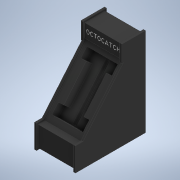
# Autodesk Inventor part: cabinet
Saved by Autodesk Inventor 2020 (Build 240168000, 168)
## iProperties
Created: 2021-03-06
Part Number: cabinet
Material: Generic
Document SubType Name: Modeling
Designer: Harry
Density: 1 g/cm^3
Appearance: Rubber - Black
Author: Harry
Autodesk Inventor part; units mm, degrees
ref_plane "YZ Plane" through (0, 0, 0) normal (1, 0, 0) x (0, 1, 0)
ref_plane "XZ Plane" through (0, 0, 0) normal (0, 1, 0) x (-1, 0, 0)
ref_plane "XY Plane" through (0, 0, 0) normal (0, 0, 1) x (1, 0, 0)
sketch "Sketch1" plane through (0, 0, 0) normal (1, 0, 0) x (0, 1, 0)
  line L0 (0, 0) -> (766.0444, -642.7876)
  line L1 (0, 0) -> (1000, 0) construction
  line L2 (0, 0) -> (0, 100)
  line L3 (0, 100) -> (-300, 100)
  line L4 (-300, 100) -> (-300, -642.7876)
  line L5 (-300, -642.7876) -> (-300, -892.7876)
  line L6 (-300, -892.7876) -> (666.0444, -892.7876)
  line L7 (666.0444, -892.7876) -> (966.0444, -892.7876)
  line L8 (966.0444, -892.7876) -> (966.0444, -592.7876)
  line L9 (966.0444, -592.7876) -> (766.0444, -592.7876)
  line L10 (766.0444, -592.7876) -> (766.0444, -642.7876)
  dimension "d0" = 1000
  dimension "d1" = 40
  dimension "d2" = 100
  dimension "d3" = 300
  dimension "d8" = 250
  dimension "d30" = 200
  dimension "d31" = 300
  constraints: 22 end point, 3 parallel, 2 horizontal, 2 perpendicular, 1 equal length, 1 vertical
  measures "d0" distance of L0.start L0.end
  measures "d1" angle of L0 L1
  measures "d2" distance of L0.start L2.end
  measures "d3" distance of L2.end L3.end
  measures "d8" distance of L4.end L5.end
  measures "d30" distance of L9.end L8.end
  measures "d31" distance of L8.end L7.end
extrude "Extrusion1" add sketch "Sketch1" against normal blind 550
sketch "Sketch3" plane through (-550, 766.0444, -642.7876) normal (0, 0.6427876, 0.7660444) x (1, 0, 0)
  line L0 (0, -1000) -> (0, 0) projected
  line L1 (550, 0) -> (550, -1000) projected
  line L2 (0, 0) -> (550, -1000) construction
  line L3 (550, -1000) -> (0, -1000) projected
  line L4 (0, -1000) -> (550, 0) construction
  line L5 (125, -760) -> (125, -240)
  line L6 (425, -240) -> (425, -760)
  line L7 (425, -760) -> (125, -240) construction
  line L8 (125, -760) -> (425, -240) construction
  line L9 (425, -240) -> (505, -240) construction
  line L10 (45, -240) -> (45, -200)
  line L11 (505, -200) -> (505, -240)
  line L12 (425, -760) -> (505, -760) construction
  line L13 (45, -760) -> (45, -800)
  line L14 (505, -800) -> (505, -760)
  line L15 (505, -760) -> (425, -760)
  line L16 (125, -760) -> (45, -760)
  line L17 (125, -240) -> (132, -240)
  line L18 (418, -240) -> (425, -240)
  line L19 (505, -240) -> (418, -240)
  line L20 (132, -240) -> (45, -240)
  line L21 (505, -800) -> (505, -910)
  line L22 (505, -910) -> (45, -910)
  line L23 (45, -910) -> (45, -800)
  line L24 (505, -200) -> (505, -100)
  line L25 (505, -100) -> (45, -100)
  line L26 (45, -100) -> (45, -200)
  point P0 (275, -500)
  dimension "d9" = 300
  dimension "d10" = 520
  dimension "d11" = 80
  dimension "d12" = 460
  dimension "d13" = 40
  dimension "d14" = 80
  dimension "d15" = 460
  dimension "d16" = 40
  dimension "d21" = 110
  dimension "d22" = 100
  constraints: 48 end point, 6 horizontal, 5 parallel, 4 midpoint, 4 perpendicular, 2 point on line
  measures "d9" distance of L5.end L6.start
  measures "d10" distance of L5.start L5.end
  measures "d11" distance of L6.start L9.end
  measures "d12" distance of L10.end L11.start
  measures "d13" distance of L10.start L10.end
  measures "d14" distance of L6.end L12.end
  measures "d15" distance of L14.start L13.end
  measures "d16" distance of L13.end L13.start
  measures "d21" distance of L21.start L21.end
  measures "d22" distance of L24.end L24.start
extrude "Extrusion3" cut sketch "Sketch3" against normal blind 130
sketch "Sketch4" plane through (-550, 682.4821, -742.3734) normal (0, 0.6427876, 0.7660444) x (1, 0, 0)
  line L0 (125, -760) -> (125, -240) projected
  line L1 (125, -240) -> (425, -760) construction
  line L2 (425, -240) -> (425, -760) projected
  line L3 (125, -760) -> (425, -240) construction
  line L4 (45, -100) -> (505, -100) projected
  line L5 (245, -900) -> (305, -900)
  line L6 (305, -900) -> (305, -100)
  line L7 (305, -100) -> (245, -100)
  line L8 (245, -100) -> (245, -900)
  line L9 (245, -900) -> (305, -100) construction
  line L10 (305, -900) -> (245, -100) construction
  point P0 (550, -1000)
  point P1 (275, -500)
  dimension "d23" = 60
  constraints: 16 end point, 3 midpoint, 2 parallel, 1 horizontal, 1 perpendicular, 1 point on line
  measures "d23" distance of L7.end L6.end
extrude "Extrusion4" cut sketch "Sketch4" against normal blind 60
sketch "Sketch5" plane through (0, 766.0444, -592.7876) normal (0, 0, 1) x (1, 0, 0)
  line L0 (-528.9661, 137.2152) -> (-20.5062, 137.2152) construction
  line L1 (-20.5062, 137.2152) -> (-20.5062, 73.6218) construction
  line L2 (-20.5062, 73.6218) -> (-528.9661, 73.6218) construction
  line L3 (-528.9661, 73.6218) -> (-528.9661, 137.2152) construction
  spline S0 degree 2 poles (-476.9874, 105.246) (-476.9874, 93.0563) (-483.1398, 83.914) knots 0 0 0 1 1 1
  spline S1 degree 2 poles (-483.1398, 83.914) (-489.9246, 73.8518) (-500.5618, 73.8518) knots 0 0 0 1 1 1
  spline S2 degree 2 poles (-500.5618, 73.8518) (-511.1991, 73.8518) (-517.9839, 84.029) knots 0 0 0 1 1 1
  spline S3 degree 2 poles (-517.9839, 84.029) (-524.0787, 93.1713) (-524.0787, 105.246) knots 0 0 0 1 1 1
  spline S4 degree 2 poles (-524.0787, 105.246) (-524.0787, 117.2632) (-518.0414, 126.1755) knots 0 0 0 1 1 1
  spline S5 degree 2 poles (-518.0414, 126.1755) (-510.9691, 136.4677) (-500.5618, 136.4677) knots 0 0 0 1 1 1
  spline S6 degree 2 poles (-500.5618, 136.4677) (-489.4646, 136.4677) (-483.5423, 126.8655) knots 0 0 0 1 1 1
  spline S7 degree 2 poles (-483.5423, 126.8655) (-476.9874, 117.4357) (-476.9874, 105.246) knots 0 0 0 1 1 1
  spline S8 degree 2 poles (-485.7272, 105.246) (-485.7272, 114.2158) (-489.0621, 119.9656) knots 0 0 0 1 1 1
  spline S9 degree 2 poles (-489.0621, 119.9656) (-493.3745, 127.6129) (-500.5618, 127.6129) knots 0 0 0 1 1 1
  spline S10 degree 2 poles (-500.5618, 127.6129) (-507.2892, 127.6129) (-511.5441, 120.4831) knots 0 0 0 1 1 1
  spline S11 degree 2 poles (-511.5441, 120.4831) (-515.339, 114.0433) (-515.339, 105.246) knots 0 0 0 1 1 1
  spline S12 degree 2 poles (-515.339, 105.246) (-515.339, 96.2187) (-513.384, 90.3539) knots 0 0 0 1 1 1
  spline S13 degree 2 poles (-513.384, 90.3539) (-507.5192, 82.7066) (-500.5618, 82.7066) knots 0 0 0 1 1 1
  spline S14 degree 2 poles (-500.5618, 82.7066) (-493.547, 82.7066) (-487.6822, 90.3539) knots 0 0 0 1 1 1
  spline S15 degree 2 poles (-487.6822, 90.3539) (-485.7272, 96.2762) (-485.7272, 105.246) knots 0 0 0 1 1 1
  spline S16 degree 2 poles (-423.3987, 83.914) (-428.3436, 77.9342) (-437.0834, 73.6218) (-443.2358, 73.6218) knots 0 0 0 1 2 2 2
  spline S17 degree 2 poles (-443.2358, 73.6218) (-453.183, 73.6218) (-465.8902, 91.2738) (-465.8902, 105.7635) knots 0 0 0 1 2 2 2
  spline S18 degree 2 poles (-465.8902, 105.7635) (-465.8902, 121.7481) (-458.3004, 130.0279) knots 0 0 0 1 1 1
  spline S19 degree 2 poles (-458.3004, 130.0279) (-452.148, 136.7552) (-443.2358, 136.7552) knots 0 0 0 1 1 1
  spline S20 degree 2 poles (-443.2358, 136.7552) (-436.5659, 136.7552) (-428.1136, 132.0403) (-424.7787, 126.003) knots 0 0 0 1 2 2 2
  spline S21 degree 2 poles (-424.7787, 126.003) (-424.2612, 125.0255) (-424.2612, 123.933) knots 0 0 0 1 1 1
  spline S22 degree 2 poles (-424.2612, 123.933) (-424.2612, 122.1506) (-427.0212, 119.5631) (-428.7461, 119.5631) knots 0 0 0 1 2 2 2
  spline S23 degree 2 poles (-428.7461, 119.5631) (-431.1611, 119.5631) (-432.426, 121.8631) knots 0 0 0 1 1 1
  spline S24 degree 2 poles (-432.426, 121.8631) (-435.8184, 127.9004) (-443.0058, 127.9004) knots 0 0 0 1 1 1
  spline S25 degree 2 poles (-443.0058, 127.9004) (-448.5256, 127.9004) (-452.2055, 123.358) knots 0 0 0 1 1 1
  spline S26 degree 2 poles (-452.2055, 123.358) (-457.0929, 117.2057) (-457.0929, 105.7635) knots 0 0 0 1 1 1
  spline S27 degree 2 poles (-457.0929, 105.7635) (-457.0929, 95.2412) (-448.8706, 82.3616) (-443.0058, 82.3616) knots 0 0 0 1 2 2 2
  spline S28 degree 2 poles (-443.0058, 82.3616) (-435.7034, 82.3616) (-430.8161, 87.5939) knots 0 0 0 1 1 1
  spline S29 degree 2 poles (-430.8161, 87.5939) (-429.2061, 90.9289) (-427.1362, 90.9289) knots 0 0 0 1 1 1
  spline S30 degree 2 poles (-427.1362, 90.9289) (-425.4112, 90.9289) (-422.5363, 88.2264) (-422.5363, 86.3865) knots 0 0 0 1 2 2 2
  spline S31 degree 2 poles (-422.5363, 86.3865) (-422.5363, 84.7765) (-423.3987, 83.914) knots 0 0 0 1 1 1
  line L4 (-370.3276, 127.5554) -> (-385.1622, 127.5554)
  line L5 (-385.1622, 127.5554) -> (-385.1622, 78.2792)
  spline S32 degree 2 poles (-385.1622, 78.2792) (-385.1622, 73.6218) (-389.6471, 73.6218) knots 0 0 0 1 1 1
  spline S33 degree 2 poles (-389.6471, 73.6218) (-394.1895, 73.6218) (-394.1895, 78.2792) knots 0 0 0 1 1 1
  line L6 (-394.1895, 78.2792) -> (-394.1895, 127.5554)
  line L7 (-394.1895, 127.5554) -> (-408.9666, 127.5554)
  spline S34 degree 2 poles (-408.9666, 127.5554) (-413.509, 127.5554) (-413.509, 132.0978) knots 0 0 0 1 1 1
  spline S35 degree 2 poles (-413.509, 132.0978) (-413.509, 136.6402) (-408.9666, 136.6402) knots 0 0 0 1 1 1
  line L8 (-408.9666, 136.6402) -> (-370.3276, 136.6402)
  spline S36 degree 2 poles (-370.3276, 136.6402) (-365.7277, 136.6402) (-365.7277, 132.0978) knots 0 0 0 1 1 1
  spline S37 degree 2 poles (-365.7277, 132.0978) (-365.7277, 127.5554) (-370.3276, 127.5554) knots 0 0 0 1 1 1
  spline S38 degree 2 poles (-310.0691, 105.246) (-310.0691, 93.0563) (-316.2214, 83.914) knots 0 0 0 1 1 1
  spline S39 degree 2 poles (-316.2214, 83.914) (-323.0062, 73.8518) (-333.6435, 73.8518) knots 0 0 0 1 1 1
  spline S40 degree 2 poles (-333.6435, 73.8518) (-344.2807, 73.8518) (-351.0655, 84.029) knots 0 0 0 1 1 1
  spline S41 degree 2 poles (-351.0655, 84.029) (-357.1604, 93.1713) (-357.1604, 105.246) knots 0 0 0 1 1 1
  spline S42 degree 2 poles (-357.1604, 105.246) (-357.1604, 117.2632) (-351.123, 126.1755) knots 0 0 0 1 1 1
  spline S43 degree 2 poles (-351.123, 126.1755) (-344.0507, 136.4677) (-333.6435, 136.4677) knots 0 0 0 1 1 1
  spline S44 degree 2 poles (-333.6435, 136.4677) (-322.5463, 136.4677) (-316.6239, 126.8655) knots 0 0 0 1 1 1
  spline S45 degree 2 poles (-316.6239, 126.8655) (-310.0691, 117.4357) (-310.0691, 105.246) knots 0 0 0 1 1 1
  spline S46 degree 2 poles (-318.8088, 105.246) (-318.8088, 114.2158) (-322.1438, 119.9656) knots 0 0 0 1 1 1
  spline S47 degree 2 poles (-322.1438, 119.9656) (-326.4562, 127.6129) (-333.6435, 127.6129) knots 0 0 0 1 1 1
  spline S48 degree 2 poles (-333.6435, 127.6129) (-340.3708, 127.6129) (-344.6257, 120.4831) knots 0 0 0 1 1 1
  spline S49 degree 2 poles (-344.6257, 120.4831) (-348.4206, 114.0433) (-348.4206, 105.246) knots 0 0 0 1 1 1
  spline S50 degree 2 poles (-348.4206, 105.246) (-348.4206, 96.2187) (-346.4657, 90.3539) knots 0 0 0 1 1 1
  spline S51 degree 2 poles (-346.4657, 90.3539) (-340.6008, 82.7066) (-333.6435, 82.7066) knots 0 0 0 1 1 1
  spline S52 degree 2 poles (-333.6435, 82.7066) (-326.6287, 82.7066) (-320.7638, 90.3539) knots 0 0 0 1 1 1
  spline S53 degree 2 poles (-320.7638, 90.3539) (-318.8088, 96.2762) (-318.8088, 105.246) knots 0 0 0 1 1 1
  spline S54 degree 2 poles (-256.4804, 83.914) (-261.4253, 77.9342) (-270.1651, 73.6218) (-276.3174, 73.6218) knots 0 0 0 1 2 2 2
  spline S55 degree 2 poles (-276.3174, 73.6218) (-286.2647, 73.6218) (-298.9718, 91.2738) (-298.9718, 105.7635) knots 0 0 0 1 2 2 2
  spline S56 degree 2 poles (-298.9718, 105.7635) (-298.9718, 121.7481) (-291.382, 130.0279) knots 0 0 0 1 1 1
  spline S57 degree 2 poles (-291.382, 130.0279) (-285.2297, 136.7552) (-276.3174, 136.7552) knots 0 0 0 1 1 1
  spline S58 degree 2 poles (-276.3174, 136.7552) (-269.6476, 136.7552) (-261.1953, 132.0403) (-257.8604, 126.003) knots 0 0 0 1 2 2 2
  spline S59 degree 2 poles (-257.8604, 126.003) (-257.3429, 125.0255) (-257.3429, 123.933) knots 0 0 0 1 1 1
  spline S60 degree 2 poles (-257.3429, 123.933) (-257.3429, 122.1506) (-260.1028, 119.5631) (-261.8278, 119.5631) knots 0 0 0 1 2 2 2
  spline S61 degree 2 poles (-261.8278, 119.5631) (-264.2427, 119.5631) (-265.5077, 121.8631) knots 0 0 0 1 1 1
  spline S62 degree 2 poles (-265.5077, 121.8631) (-268.9001, 127.9004) (-276.0874, 127.9004) knots 0 0 0 1 1 1
  spline S63 degree 2 poles (-276.0874, 127.9004) (-281.6073, 127.9004) (-285.2872, 123.358) knots 0 0 0 1 1 1
  spline S64 degree 2 poles (-285.2872, 123.358) (-290.1746, 117.2057) (-290.1746, 105.7635) knots 0 0 0 1 1 1
  spline S65 degree 2 poles (-290.1746, 105.7635) (-290.1746, 95.2412) (-281.9523, 82.3616) (-276.0874, 82.3616) knots 0 0 0 1 2 2 2
  spline S66 degree 2 poles (-276.0874, 82.3616) (-268.7851, 82.3616) (-263.8977, 87.5939) knots 0 0 0 1 1 1
  spline S67 degree 2 poles (-263.8977, 87.5939) (-262.2877, 90.9289) (-260.2178, 90.9289) knots 0 0 0 1 1 1
  spline S68 degree 2 poles (-260.2178, 90.9289) (-258.4928, 90.9289) (-255.6179, 88.2264) (-255.6179, 86.3865) knots 0 0 0 1 2 2 2
  spline S69 degree 2 poles (-255.6179, 86.3865) (-255.6179, 84.7765) (-256.4804, 83.914) knots 0 0 0 1 1 1
  spline S70 degree 2 poles (-193.8644, 79.8316) (-193.577, 78.9692) (-193.577, 78.1642) knots 0 0 0 1 1 1
  spline S71 degree 2 poles (-193.577, 78.1642) (-193.577, 76.2667) (-196.4519, 73.8518) (-198.1768, 73.8518) knots 0 0 0 1 2 2 2
  spline S72 degree 2 poles (-198.1768, 73.8518) (-201.1093, 73.8518) (-202.0867, 76.6117) knots 0 0 0 1 1 1
  line L9 (-202.0867, 76.6117) -> (-205.6517, 85.294)
  line L10 (-205.6517, 85.294) -> (-233.711, 85.294)
  line L11 (-233.711, 85.294) -> (-236.9884, 76.6692)
  spline S73 degree 2 poles (-236.9884, 76.6692) (-238.1958, 73.8518) (-241.1283, 73.8518) knots 0 0 0 1 1 1
  spline S74 degree 2 poles (-241.1283, 73.8518) (-245.5557, 73.8518) (-245.5557, 78.1067) knots 0 0 0 1 1 1
  spline S75 degree 2 poles (-245.5557, 78.1067) (-245.5557, 78.9117) (-245.3257, 79.6016) knots 0 0 0 1 1 1
  line L12 (-245.3257, 79.6016) -> (-224.5112, 134.5128)
  spline S76 degree 2 poles (-224.5112, 134.5128) (-222.7287, 137.2152) (-220.0838, 137.2152) knots 0 0 0 1 1 1
  spline S77 degree 2 poles (-220.0838, 137.2152) (-217.4389, 137.2152) (-215.5989, 134.5703) knots 0 0 0 1 1 1
  line L13 (-215.5989, 134.5703) -> (-193.8644, 79.8316)
  line L14 (-208.5841, 94.0338) -> (-219.9688, 123.9905)
  line L15 (-219.9688, 123.9905) -> (-231.0085, 94.0338)
  line L16 (-231.0085, 94.0338) -> (-208.5841, 94.0338)
  line L17 (-139.8733, 127.5554) -> (-154.7079, 127.5554)
  line L18 (-154.7079, 127.5554) -> (-154.7079, 78.2792)
  spline S78 degree 2 poles (-154.7079, 78.2792) (-154.7079, 73.6218) (-159.1928, 73.6218) knots 0 0 0 1 1 1
  spline S79 degree 2 poles (-159.1928, 73.6218) (-163.7352, 73.6218) (-163.7352, 78.2792) knots 0 0 0 1 1 1
  line L19 (-163.7352, 78.2792) -> (-163.7352, 127.5554)
  line L20 (-163.7352, 127.5554) -> (-178.5123, 127.5554)
  spline S80 degree 2 poles (-178.5123, 127.5554) (-183.0547, 127.5554) (-183.0547, 132.0978) knots 0 0 0 1 1 1
  spline S81 degree 2 poles (-183.0547, 132.0978) (-183.0547, 136.6402) (-178.5123, 136.6402) knots 0 0 0 1 1 1
  line L21 (-178.5123, 136.6402) -> (-139.8733, 136.6402)
  spline S82 degree 2 poles (-139.8733, 136.6402) (-135.2734, 136.6402) (-135.2734, 132.0978) knots 0 0 0 1 1 1
  spline S83 degree 2 poles (-135.2734, 132.0978) (-135.2734, 127.5554) (-139.8733, 127.5554) knots 0 0 0 1 1 1
  spline S84 degree 2 poles (-82.3172, 83.914) (-87.2621, 77.9342) (-96.0019, 73.6218) (-102.1542, 73.6218) knots 0 0 0 1 2 2 2
  spline S85 degree 2 poles (-102.1542, 73.6218) (-112.1015, 73.6218) (-124.8087, 91.2738) (-124.8087, 105.7635) knots 0 0 0 1 2 2 2
  spline S86 degree 2 poles (-124.8087, 105.7635) (-124.8087, 121.7481) (-117.2189, 130.0279) knots 0 0 0 1 1 1
  spline S87 degree 2 poles (-117.2189, 130.0279) (-111.0665, 136.7552) (-102.1542, 136.7552) knots 0 0 0 1 1 1
  spline S88 degree 2 poles (-102.1542, 136.7552) (-95.4844, 136.7552) (-87.0321, 132.0403) (-83.6972, 126.003) knots 0 0 0 1 2 2 2
  spline S89 degree 2 poles (-83.6972, 126.003) (-83.1797, 125.0255) (-83.1797, 123.933) knots 0 0 0 1 1 1
  spline S90 degree 2 poles (-83.1797, 123.933) (-83.1797, 122.1506) (-85.9396, 119.5631) (-87.6646, 119.5631) knots 0 0 0 1 2 2 2
  spline S91 degree 2 poles (-87.6646, 119.5631) (-90.0795, 119.5631) (-91.3445, 121.8631) knots 0 0 0 1 1 1
  spline S92 degree 2 poles (-91.3445, 121.8631) (-94.7369, 127.9004) (-101.9242, 127.9004) knots 0 0 0 1 1 1
  spline S93 degree 2 poles (-101.9242, 127.9004) (-107.4441, 127.9004) (-111.124, 123.358) knots 0 0 0 1 1 1
  spline S94 degree 2 poles (-111.124, 123.358) (-116.0114, 117.2057) (-116.0114, 105.7635) knots 0 0 0 1 1 1
  spline S95 degree 2 poles (-116.0114, 105.7635) (-116.0114, 95.2412) (-107.7891, 82.3616) (-101.9242, 82.3616) knots 0 0 0 1 2 2 2
  spline S96 degree 2 poles (-101.9242, 82.3616) (-94.6219, 82.3616) (-89.7345, 87.5939) knots 0 0 0 1 1 1
  spline S97 degree 2 poles (-89.7345, 87.5939) (-88.1246, 90.9289) (-86.0546, 90.9289) knots 0 0 0 1 1 1
  spline S98 degree 2 poles (-86.0546, 90.9289) (-84.3297, 90.9289) (-81.4547, 88.2264) (-81.4547, 86.3865) knots 0 0 0 1 2 2 2
  spline S99 degree 2 poles (-81.4547, 86.3865) (-81.4547, 84.7765) (-82.3172, 83.914) knots 0 0 0 1 1 1
  spline S100 degree 2 poles (-26.6586, 78.3942) (-26.6586, 73.8518) (-31.0285, 73.8518) knots 0 0 0 1 1 1
  spline S101 degree 2 poles (-31.0285, 73.8518) (-35.4559, 73.8518) (-35.4559, 78.3942) knots 0 0 0 1 1 1
  line L22 (-35.4559, 78.3942) -> (-35.4559, 102.7736)
  line L23 (-35.4559, 102.7736) -> (-61.3877, 102.7736)
  line L24 (-61.3877, 102.7736) -> (-61.3877, 78.3942)
  spline S102 degree 2 poles (-61.3877, 78.3942) (-61.3877, 73.8518) (-65.8726, 73.8518) knots 0 0 0 1 1 1
  spline S103 degree 2 poles (-65.8726, 73.8518) (-70.3, 73.8518) (-70.3, 78.3942) knots 0 0 0 1 1 1
  line L25 (-70.3, 78.3942) -> (-70.3, 132.2128)
  spline S104 degree 2 poles (-70.3, 132.2128) (-70.3, 136.7552) (-65.8726, 136.7552) knots 0 0 0 1 1 1
  spline S105 degree 2 poles (-65.8726, 136.7552) (-61.3877, 136.7552) (-61.3877, 132.2128) knots 0 0 0 1 1 1
  line L26 (-61.3877, 132.2128) -> (-61.3877, 111.6283)
  line L27 (-61.3877, 111.6283) -> (-35.4559, 111.6283)
  line L28 (-35.4559, 111.6283) -> (-35.4559, 132.2128)
  spline S106 degree 2 poles (-35.4559, 132.2128) (-35.4559, 136.7552) (-31.0285, 136.7552) knots 0 0 0 1 1 1
  spline S107 degree 2 poles (-31.0285, 136.7552) (-26.6586, 136.7552) (-26.6586, 132.2128) knots 0 0 0 1 1 1
  line L29 (-26.6586, 132.2128) -> (-26.6586, 78.3942)
  point P0 (0, -766.0444)
  constraints: 2 other
extrude "Extrusion5" add sketch "Sketch5" along normal blind 3
sketch "Sketch6" plane through (0, 0, 0) normal (1, 0, 0) x (0, 0, -1)
  line L0 (567.7876, 991.0444) -> (917.7876, 991.0444)
  line L1 (917.7876, 991.0444) -> (917.7876, -325)
  line L2 (917.7876, -325) -> (-125, -325)
  line L3 (-125, -325) -> (-125, 25)
  line L4 (-125, 25) -> (-11.6577, 25)
  line L5 (-11.6577, 25) -> (589.1749, 741.0444)
  line L6 (589.1749, 741.0444) -> (567.7876, 741.0444)
  line L7 (567.7876, 741.0444) -> (567.7876, 991.0444)
  point P0 (0, 0)
  constraints: 16 end point
extrude "Extrusion6" add sketch "Sketch6" along normal blind 30
ref_plane "Work Plane1" through (-275, 0, 0) normal (1, 0, 0) x (0, 0, -1)
mirror "Mirror1" about plane through (-275, 0, 0) normal (1, 0, 0) of "Extrusion6"
body "Solid1"
